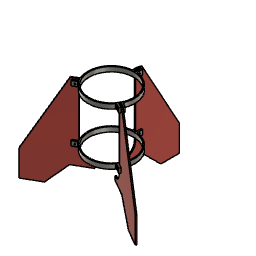
Large Rocket Fin Assembly v2 (Autodesk Fusion 360 design; units mm, degrees)
Autodesk Fusion 360 part; units mm, degrees
sketch "Sketch1" plane through (0, 0, 0) normal (0, 0, 1) x (1, 0, 0)
  circle A0 centre (0, 0) radius 30.48
  line L0 (0, 30.48) -> (0, 31.877)
  line L1 (0, 31.877) -> (0, 32.512)
  line L2 (-1.016, 39.497) -> (-3.175, 39.497)
  line L3 (1.016, 39.497) -> (3.175, 39.497)
  line L4 (3.175, 39.497) -> (3.175, 31.7185)
  line L5 (-3.175, 39.497) -> (-3.175, 31.7185)
  line L6 (-1.016, 39.497) -> (-1.016, 32.512)
  line L7 (-1.016, 32.512) -> (1.016, 32.512)
  line L8 (1.016, 32.512) -> (1.016, 39.497)
  line L9 (-33.6974, -20.6284) -> (-27.6482, -17.1359)
  line L10 (-32.6179, -22.4981) -> (-25.8815, -18.6089)
  line L11 (-28.6642, -15.3761) -> (-34.7134, -18.8686)
  line L12 (-35.7929, -16.9989) -> (-29.0565, -13.1096)
  line L13 (-34.7134, -18.8686) -> (-35.7929, -16.9989)
  line L14 (-33.6974, -20.6284) -> (-32.6179, -22.4981)
  line L15 (-27.6482, -17.1359) -> (-28.6642, -15.3761)
  line L16 (34.7134, -18.8686) -> (28.6642, -15.3761)
  line L17 (35.7929, -16.9989) -> (29.0565, -13.1096)
  line L18 (27.6482, -17.1359) -> (33.6974, -20.6284)
  line L19 (32.6179, -22.4981) -> (25.8815, -18.6089)
  line L20 (33.6974, -20.6284) -> (32.6179, -22.4981)
  line L21 (34.7134, -18.8686) -> (35.7929, -16.9989)
  line L22 (28.6642, -15.3761) -> (27.6482, -17.1359)
  arc A1 (-3.175, 31.7185) -> (-29.0565, -13.1096) centre (0, 0) ccw
  arc A2 (-25.8815, -18.6089) -> (25.8815, -18.6089) centre (0, 0) ccw
  arc A3 (29.0565, -13.1096) -> (3.175, 31.7185) centre (0, 0) ccw
  dimension "d2" = 60.96
  dimension "d13" = 2.032
  dimension "d15" = 360
  constraint coincident A0.centre A1.centre
  constraint vertical L0
  constraint coincident A0 L0.start
  constraint parallel L0 L1
  constraint perpendicular L1 L2
  constraint perpendicular L1 L3
  constraint perpendicular L3 L4
  constraint coincident L5.end A2
  constraint perpendicular L2 L6
  constraint perpendicular L1 L7
  constraint perpendicular L3 L8
  constraint coincident L7 L1.end
  constraint concentric A0 A2
  constraint concentric A1 A2
  constraint concentric A2 A3
  measures "d2" diameter of A0
  measures "d13" distance of L6.end L7.end
extrude "Extrude1" add sketch "Sketch1" along normal blind 6.35 makes body 1
sketch "Sketch2" plane through (3.175, 0, 0) normal (1, 0, 0) x (0, 1, 0)
  line L0 (31.7185, 0) -> (39.497, 0)
  line L1 (39.497, 0) -> (39.497, 6.35)
  line L2 (39.497, 6.35) -> (31.7185, 6.35)
  line L3 (31.7185, 6.35) -> (31.7185, 0)
  circle A0 centre (35.56, 3.302) radius 0.9525
  dimension "d18" = 1.905
  measures "d18" diameter of A0
extrude "Extrude2" cut sketch "Sketch2" against normal blind 19.05 contours A0 bodies 1
sketch "Sketch3" plane through (-1.5875, -2.7496, 0) normal (-0.5, -0.866025, 0) x (0.866025, -0.5, 0)
  line L0 (31.7185, 0) -> (39.497, 0)
  line L1 (39.497, 0) -> (39.497, 6.35)
  line L2 (39.497, 6.35) -> (31.7185, 6.35)
  line L3 (31.7185, 6.35) -> (31.7185, 0)
  circle A0 centre (35.56, 3.048) radius 0.9525
  dimension "d21" = 1.905
  measures "d21" diameter of A0
extrude "Extrude3" cut sketch "Sketch3" against normal blind 33.02 contours A0 bodies 1
sketch "Sketch4" plane through (1.5875, -2.7496, 0) normal (0.5, -0.866025, 0) x (0.866025, 0.5, 0)
  line L0 (-39.497, 0) -> (-31.7185, 0)
  line L1 (-31.7185, 0) -> (-31.7185, 6.35)
  line L2 (-31.7185, 6.35) -> (-39.497, 6.35)
  line L3 (-39.497, 6.35) -> (-39.497, 0)
  circle A0 centre (-35.56, 3.048) radius 0.9525
  dimension "d24" = 1.905
  measures "d24" diameter of A0
extrude "Extrude4" cut sketch "Sketch4" against normal blind 16.51 contours A0 bodies 1
ref_plane "WorkPlane1" through (31.5618, -17.3423, 3.175) normal (-0.5, -0.866025, 0) x (0.866025, -0.5, 0)
sketch "Sketch5" plane through (31.5618, -17.3423, 3.175) normal (-0.5, -0.866025, 0) x (0.866025, -0.5, 0)
  line L0 (-3.6818, 4.812) -> (-3.6818, -79.008)
  arc A0 (-19.8655, -93.2601) -> (-3.6818, -79.008) centre (-18.5819, -78.403) ccw
  line L1 (-19.8655, -93.2601) -> (-19.8655, -98.3401)
  line L2 (-19.8655, -98.3401) -> (5.5345, -98.3401)
  line L3 (5.5345, -98.3401) -> (30.6792, -123.4848)
  line L4 (5.5345, -98.3401) -> (30.9345, -98.3401) construction
  line L5 (30.6792, -123.4848) -> (56.0792, -123.4848)
  line L6 (56.0792, -123.4848) -> (56.0792, -87.9248)
  line L7 (-3.6818, 4.812) -> (5.08, 4.812)
  line L8 (5.08, 4.812) -> (56.0792, -87.9248)
  dimension "d28" = 83.82
  dimension "d30" = 21.5646
  dimension "d31" = 5.08
  dimension "d32" = 25.4
  dimension "d33" = 45
  dimension "d34" = 35.56
  dimension "d35" = 25.4
  dimension "d36" = 35.56
  constraint vertical L0
  constraint vertical L1
  constraint perpendicular L1 L2
  constraint horizontal L4
  constraint horizontal L5
  constraint perpendicular L5 L6
  constraint perpendicular L0 L7
  measures "d28" distance of L0.start L0.end
  measures "d30" distance of L0.end A0.start
  measures "d31" distance of A0.start L1.end
  measures "d32" distance of L1.end L2.end
  measures "d33" angle of L3 L4
  measures "d34" distance of L2.end L3.end
  measures "d35" distance of L3.end L5.end
  measures "d36" distance of L5.end L6.end
extrude "Extrude5" add sketch "Sketch5" along normal blind 1.524 separate body makes body 2
pattern_circular "C-Pattern1" count 3 over 360 about axis through (0, 0, 0) along (0, 0, 1) of bodies 2 makes body 3 at (-0.762, 55.1636, -50.8653) makes body 4 at (-47.3921, -28.2417, -50.8653)
copy_body "CopyPasteBodies1" bodies 1 makes body 5
move_body "Move1" bodies 5 to x (1, 0, 0) y (0, 1, 0) z (0, 0, 1) at (0, 0, -71.12)
hole "Hole1" at (-3.175, 35.56, -67.818) direction (1, 0, 0) diameter 1.778 depth 7.62 tip angle 180 bodies 3
thread "Thread1" "ANSI Unified Screw Threads 0.086(#2) 2-56 UNC 3B"
hole "Hole2" at (-29.2084, -20.5296, -68.072) direction (-0.5, 0.866025, 0) diameter 1.778 depth 7.62 tip angle 180 bodies 4
thread "Thread2" "ANSI Unified Screw Threads 0.086(#2) 2-56 UNC 3B"
hole "Hole3" at (29.2084, -20.5296, -68.072) direction (0.5, 0.866025, 0) diameter 1.778 depth 7.62 tip angle 180 bodies 2
thread "Thread3" "ANSI Unified Screw Threads 0.086(#2) 2-56 UNC 3B"
hole "Hole4" at (-29.2084, -20.5296, 3.048) direction (-0.5, 0.866025, 0) diameter 1.778 depth 7.62 tip angle 180 bodies 4
thread "Thread4" "ANSI Unified Screw Threads 0.086(#2) 2-56 UNC 3B"
hole "Hole5" at (29.2084, -20.5296, 3.048) direction (0.5, 0.866025, 0) diameter 1.778 depth 7.62 tip angle 180 bodies 2
thread "Thread5" "ANSI Unified Screw Threads 0.086(#2) 2-56 UNC 3B"
hole "Hole6" at (3.175, 35.56, 3.302) direction (-1, 0, 0) diameter 1.778 depth 7.62 tip angle 180 bodies 3
thread "Thread6" "ANSI Unified Screw Threads 0.086(#2) 2-56 UNC 3B"
fillet "Fillet1" radius 1.27 12 edges at (-3.175, 31.7185, 3.175) (-29.0565, -13.1096, 3.175) (25.8815, -18.6089, 3.175) (-25.8815, -18.6089, 3.175) (3.175, 31.7185, 3.175) (29.0565, -13.1096, 3.175) (-3.175, 31.7185, -67.945) (-29.0565, -13.1096, -67.945) (25.8815, -18.6089, -67.945) (-25.8815, -18.6089, -67.945) (29.0565, -13.1096, -67.945) (3.175, 31.7185, -67.945) on bodies 1 5
